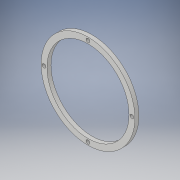
# Autodesk Inventor part: ベアリング 外側
Saved by Autodesk Inventor 2019 (Build 230136000, 136)
## iProperties
Created: 2020-09-30
Part Number: ベアリング 外側
Material: 一般
Document SubType Name: Modeling
Designer: Toshihito
Density: 1 g/cm^3
Appearance: 既定
Author: Toshihito
Autodesk Inventor part; units mm, degrees
ref_plane "YZ Plane" through (0, 0, 0) normal (1, 0, 0) x (0, 1, 0)
ref_plane "XZ Plane" through (0, 0, 0) normal (0, 1, 0) x (-1, 0, 0)
ref_plane "XY Plane" through (0, 0, 0) normal (0, 0, 1) x (1, 0, 0)
sketch "スケッチ1" plane through (0, 0, 0) normal (0, 0, 1) x (1, 0, 0)
  circle A0 centre (0, 0) radius 87.5
  circle A1 centre (0, 0) radius 100
  circle A2 centre (0, 0) radius 93.75 construction
  circle A3 centre (0, 93.75) radius 4
  circle A4 centre (93.75, 0) radius 4
  circle A5 centre (0, -93.75) radius 4
  circle A6 centre (-93.75, 0) radius 4
  dimension "d0" = 175
  dimension "d1" = 200
  dimension "d2" = 187.5
  dimension "d3" = 8
  dimension "d4" = 8
  dimension "d5" = 8
  dimension "d6" = 8
  constraints: 7 centre point, 4 point on circle, 3 coincident
  measures "d0" diameter of A0
  measures "d1" diameter of A1
  measures "d2" diameter of A2
  measures "d3" diameter of A3
  measures "d4" diameter of A4
  measures "d5" diameter of A5
  measures "d6" diameter of A6
extrude "押し出し1" add sketch "スケッチ1" along normal blind 8.5
